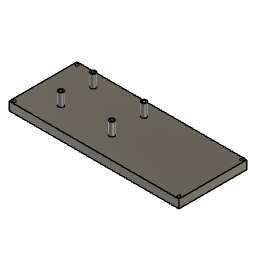
achterkant (Autodesk Fusion 360 design; units mm, degrees)
Autodesk Fusion 360 part; units mm, degrees
sketch "Sketch1" plane through (0, 0, 0) normal (0, 0, 1) x (1, 0, 0)
  line L0 (-25, 50) -> (175, 50)
  line L1 (175, 50) -> (175, -30)
  line L2 (175, -30) -> (-25, -30)
  line L3 (-25, -30) -> (-25, 50)
  constraint horizontal L0
  constraint vertical L1
  constraint horizontal L2
  constraint vertical L3
extrude "Extrude1" add sketch "Sketch1" along normal blind 10
sketch "Sketch2" plane through (0, 0, 35) normal (0, 0, 1) x (1, 0, 0)
  line L0 (10, 34, -30) -> (70, 34, -30)
  line L1 (70, 34, -30) -> (70, -4, -30)
  line L2 (70, -4, -30) -> (10, -4, -30)
  line L3 (10, -4, -30) -> (10, 34, -30)
  circle A0 through (13, 34, -30) (8.5, 36.5981, -30) (8.5, 31.4019, -30)
  circle A1 through (73, 34, -30) (68.5, 36.5981, -30) (68.5, 31.4019, -30)
  circle A2 through (13, -4, -30) (8.5, -1.4019, -30) (8.5, -6.5981, -30)
  circle A3 through (73, -4, -30) (68.5, -1.4019, -30) (68.5, -6.5981, -30)
  dimension "d99" = 6
  dimension "d100" = 6
  dimension "d101" = 6
  dimension "d102" = 6
extrude "Extrude2" add sketch "Sketch2" along normal blind 20 contours L0 L3 A0 | L0 L3 A0 | L0 L1 A1 | L0 L1 A1 | L2 L3 A2 | L2 L3 A2 | L1 L2 A3 | L1 L2 A3 in plane through (0, 0, 5) normal (0, 0, 1)
hole "Hole1" at (10, 34, 25) direction (0, 0, -1) diameter 3.332 depth 12 tip angle 180
thread "Thread1" "ISO Metric profile 4.0 M4x0.7 6H" major diameter 4.1095 minor diameter 3.332 pitch 0.7 angle 60 resizes the face on face at (10.083, 32.3361, 21)
hole "Hole2" at (70, 34, 25) direction (0, 0, -1) diameter 3.332 depth 12 tip angle 180
thread "Thread2" "ISO Metric profile 4.0 M4x0.7 6H" major diameter 4.1095 minor diameter 3.332 pitch 0.7 angle 60 resizes the face on face at (71.2491, 35.1024, 21)
hole "Hole3" at (69.7479, -3.4249, 25) direction (0, 0, -1) diameter 3.332 depth 12 tip angle 180
thread "Thread3" "ISO Metric profile 4.0 M4x0.7 6H" major diameter 4.1095 minor diameter 3.332 pitch 0.7 angle 60 resizes the face on face at (70.8188, -2.1486, 21)
hole "Hole4" at (10, -4, 25) direction (0, 0, -1) diameter 3.332 depth 12 tip angle 180
thread "Thread4" "ISO Metric profile 4.0 M4x0.7 6H" major diameter 4.1095 minor diameter 3.332 pitch 0.7 angle 60 resizes the face on face at (10.083, -5.6639, 21)
sketch "Sketch3" plane through (0, 0, 0) normal (0, 0, -1) x (1, 0, 0)
  line L0 (175, 30) -> (-25, 30)
  line L1 (-25, 30) -> (-25, -50)
  line L2 (-25, -50) -> (175, -50)
  line L3 (175, -50) -> (175, 30)
  line L4 (-25, 30) -> (-25, 27) construction
  line L5 (-25, 27) -> (-22, 27) construction
  line L6 (75, 30) -> (75, 13) construction
  line L7 (-25, -10) -> (10, -10) construction
  point P0 (172, 27)
  point P1 (-22, -47)
  point P2 (172, -47)
  dimension "d136" = 3
  dimension "d137" = 3
  constraint coincident L0.end L1.start
  constraint perpendicular L0 L4
  constraint perpendicular L4 L5
  constraint midpoint L0 L6.start
  constraint perpendicular L0 L6
  constraint midpoint L1 L7.start
  constraint perpendicular L1 L7
  constraint symmetric L5.end L6 P0
  constraint symmetric L5.end L7 P1
  constraint symmetric L7 P0 P2
  measures "d136" distance of L0.end L4.end
  measures "d137" distance of L4.end L5.end
hole "Hole5" at (-22, -27, 0) direction (0, 0, 1) diameter 3.332 depth 22 tip angle 180
thread "Thread5" "ISO Metric profile 4.0 M4x0.7 6H" major diameter 4.1095 minor diameter 3.332 pitch 0.7 angle 60 resizes the face on face at (-23.0709, -28.2762, 3.3333)
hole "Hole6" at (172, -27, 0) direction (0, 0, 1) diameter 3.332 depth 22 tip angle 180
thread "Thread6" "ISO Metric profile 4.0 M4x0.7 6H" major diameter 4.1095 minor diameter 3.332 pitch 0.7 angle 60 resizes the face on face at (172.083, -25.3361, 3.3333)
hole "Hole7" at (172, 47, 0) direction (0, 0, 1) diameter 3.332 depth 20 tip angle 180
thread "Thread7" "ISO Metric profile 4.0 M4x0.7 6H" major diameter 4.1095 minor diameter 3.332 pitch 0.7 angle 60 resizes the face on face at (170.9941, 48.328, 3.3333)
hole "Hole8" at (-22, 47, 0) direction (0, 0, 1) diameter 3.332 depth 30 tip angle 180
thread "Thread8" "ISO Metric profile 4.0 M4x0.7 6H" major diameter 4.1095 minor diameter 3.332 pitch 0.7 angle 60 resizes the face on face at (-21.917, 48.6639, 3.3333)
